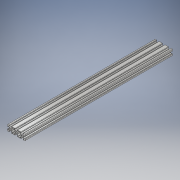
# Autodesk Inventor part: Aluminium Profile 2060 500mm
Saved by Autodesk Inventor 2019 (Build 230136000, 136)
## iProperties
Created: 2020-11-22
Part Number: Aluminium Profile 2060 500mm
Material: Aluminum 6061
Document SubType Name: Modeling
Designer: asus
Density: 2.7 g/cm^3
Appearance: Aluminum - Polished
Author: asus
Autodesk Inventor part; units mm, degrees
ref_plane "YZ Plane" through (0, 0, 0) normal (1, 0, 0) x (0, 1, 0)
ref_plane "XZ Plane" through (0, 0, 0) normal (0, 1, 0) x (-1, 0, 0)
ref_plane "XY Plane" through (0, 0, 0) normal (0, 0, 1) x (1, 0, 0)
sketch "Sketch1" plane through (0, 0, 0) normal (0, 0, 1) x (1, 0, 0)
  line L0 (-33.69, 10) -> (-33.9, 10.21)
  line L1 (-33.9, 10.21) -> (-33.9, 12.8393)
  line L2 (-33.9, 12.8393) -> (-36.5607, 15.5)
  line L3 (-36.5607, 15.5) -> (-38.2, 15.5)
  line L4 (-38.2, 15.5) -> (-38.2, 13.395)
  line L5 (-38.2, 13.395) -> (-38.815, 13.395)
  line L6 (-38.815, 13.395) -> (-40, 14.58)
  line L7 (-40, 14.58) -> (-40, 18.5)
  arc A0 (-38.5, 20) -> (-40, 18.5) centre (-38.5, 18.5) ccw
  line L8 (-38.5, 20) -> (-34.58, 20)
  line L9 (-34.58, 20) -> (-33.395, 18.815)
  line L10 (-33.395, 18.815) -> (-33.395, 18.2)
  line L11 (-33.395, 18.2) -> (-35.5, 18.2)
  line L12 (-35.5, 18.2) -> (-35.5, 16.5607)
  line L13 (-35.5, 16.5607) -> (-32.8393, 13.9)
  line L14 (-32.8393, 13.9) -> (-30.21, 13.9)
  line L15 (-30.21, 13.9) -> (-30, 13.69)
  line L16 (-30, 13.69) -> (-29.79, 13.9)
  line L17 (-29.79, 13.9) -> (-27.1607, 13.9)
  line L18 (-27.1607, 13.9) -> (-24.5, 16.5607)
  line L19 (-24.5, 16.5607) -> (-24.5, 18.2)
  line L20 (-24.5, 18.2) -> (-26.605, 18.2)
  line L21 (-26.605, 18.2) -> (-26.605, 18.815)
  line L22 (-26.605, 18.815) -> (-25.42, 20)
  line L23 (-25.42, 20) -> (-14.58, 20)
  line L24 (-14.58, 20) -> (-13.395, 18.815)
  line L25 (-13.395, 18.815) -> (-13.395, 18.2)
  line L26 (-13.395, 18.2) -> (-15.5, 18.2)
  line L27 (-15.5, 18.2) -> (-15.5, 16.5607)
  line L28 (-15.5, 16.5607) -> (-12.8393, 13.9)
  line L29 (-12.8393, 13.9) -> (-10.21, 13.9)
  line L30 (-10.21, 13.9) -> (-10, 13.69)
  line L31 (-17.3, 16.2393) -> (-17.3, 18.2)
  line L32 (-17.3, 18.2) -> (-22.7, 18.2)
  line L33 (-22.7, 18.2) -> (-22.7, 16.2393)
  line L34 (-22.7, 16.2393) -> (-26.1, 12.8393)
  line L35 (-26.1, 12.8393) -> (-26.1, 10)
  line L36 (-13.9, 10) -> (-13.9, 12.8393)
  line L37 (-13.9, 12.8393) -> (-17.3, 16.2393)
  circle A1 centre (-10, 10) radius 2.3
  circle A2 centre (-30, 10) radius 2.3
  line L38 (-24.5, 1.8) -> (-26.605, 1.8)
  line L39 (-24.5, 3.4393) -> (-24.5, 1.8)
  line L40 (-22.7, 3.7607) -> (-26.1, 7.1607)
  line L41 (-22.7, 1.8) -> (-22.7, 3.7607)
  line L42 (-29.79, 6.1) -> (-27.1607, 6.1)
  line L43 (-30, 6.31) -> (-29.79, 6.1)
  line L44 (-30.21, 6.1) -> (-30, 6.31)
  line L45 (-32.8393, 6.1) -> (-30.21, 6.1)
  line L46 (-33.9, 9.79) -> (-33.9, 7.1607)
  line L47 (-33.69, 10) -> (-33.9, 9.79)
  line L48 (-26.1, 7.1607) -> (-26.1, 10)
  line L49 (-27.1607, 6.1) -> (-24.5, 3.4393)
  line L50 (-13.9, 10) -> (-13.9, 7.1607)
  line L51 (-12.8393, 6.1) -> (-10.21, 6.1)
  line L52 (-10.21, 6.1) -> (-10, 6.31)
  line L53 (-33.395, 1.185) -> (-33.395, 1.8)
  line L54 (-35.5, 3.4393) -> (-32.8393, 6.1)
  line L55 (-33.395, 1.8) -> (-35.5, 1.8)
  line L56 (-35.5, 1.8) -> (-35.5, 3.4393)
  line L57 (-34.58, 0) -> (-33.395, 1.185)
  line L58 (-33.9, 7.1607) -> (-36.5607, 4.5)
  line L59 (-36.5607, 4.5) -> (-38.2, 4.5)
  line L60 (-38.2, 4.5) -> (-38.2, 6.605)
  line L61 (-38.2, 6.605) -> (-38.815, 6.605)
  line L62 (-38.815, 6.605) -> (-40, 5.42)
  line L63 (-38.5, 0) -> (-34.58, 0)
  arc A3 (-40, 1.5) -> (-38.5, 0) centre (-38.5, 1.5) ccw
  line L64 (-40, 5.42) -> (-40, 1.5)
  line L65 (-26.605, 1.8) -> (-26.605, 1.185)
  line L66 (-13.9, 7.1607) -> (-17.3, 3.7607)
  line L67 (-13.395, 1.8) -> (-15.5, 1.8)
  line L68 (-17.3, 3.7607) -> (-17.3, 1.8)
  line L69 (-15.5, 1.8) -> (-15.5, 3.4393)
  line L70 (-13.395, 1.185) -> (-13.395, 1.8)
  line L71 (-14.58, 0) -> (-13.395, 1.185)
  line L72 (-17.3, 1.8) -> (-22.7, 1.8)
  line L73 (-25.42, 0) -> (-14.58, 0)
  line L74 (-26.605, 1.185) -> (-25.42, 0)
  line L75 (-15.5, 3.4393) -> (-12.8393, 6.1)
  line L76 (4.5, 18.2) -> (6.605, 18.2)
  line L77 (4.5, 16.5607) -> (4.5, 18.2)
  line L78 (2.7, 16.2393) -> (6.1, 12.8393)
  line L79 (2.7, 18.2) -> (2.7, 16.2393)
  line L80 (9.79, 13.9) -> (7.1607, 13.9)
  line L81 (10, 13.69) -> (9.79, 13.9)
  line L82 (10.21, 13.9) -> (10, 13.69)
  line L83 (12.8393, 13.9) -> (10.21, 13.9)
  line L84 (13.9, 10.21) -> (13.9, 12.8393)
  line L85 (13.69, 10) -> (13.9, 10.21)
  line L86 (6.1, 12.8393) -> (6.1, 10)
  circle A4 centre (10, 10) radius 2.3
  line L87 (7.1607, 13.9) -> (4.5, 16.5607)
  line L88 (-6.1, 10) -> (-6.1, 12.8393)
  line L89 (-7.1607, 13.9) -> (-9.79, 13.9)
  line L90 (-9.79, 13.9) -> (-10, 13.69)
  line L91 (13.395, 18.815) -> (13.395, 18.2)
  line L92 (15.5, 16.5607) -> (12.8393, 13.9)
  line L93 (13.395, 18.2) -> (15.5, 18.2)
  line L94 (15.5, 18.2) -> (15.5, 16.5607)
  line L95 (14.58, 20) -> (13.395, 18.815)
  line L96 (13.9, 12.8393) -> (16.5607, 15.5)
  line L97 (16.5607, 15.5) -> (18.2, 15.5)
  line L98 (18.2, 15.5) -> (18.2, 13.395)
  line L99 (18.2, 13.395) -> (18.815, 13.395)
  line L100 (18.815, 13.395) -> (20, 14.58)
  line L101 (18.5, 20) -> (14.58, 20)
  arc A5 (20, 18.5) -> (18.5, 20) centre (18.5, 18.5) ccw
  line L102 (20, 14.58) -> (20, 18.5)
  line L103 (6.605, 18.2) -> (6.605, 18.815)
  line L104 (-6.1, 12.8393) -> (-2.7, 16.2393)
  line L105 (-6.605, 18.2) -> (-4.5, 18.2)
  line L106 (-2.7, 16.2393) -> (-2.7, 18.2)
  line L107 (-4.5, 18.2) -> (-4.5, 16.5607)
  line L108 (-6.605, 18.815) -> (-6.605, 18.2)
  line L109 (-5.42, 20) -> (-6.605, 18.815)
  line L110 (-2.7, 18.2) -> (2.7, 18.2)
  line L111 (5.42, 20) -> (-5.42, 20)
  line L112 (6.605, 18.815) -> (5.42, 20)
  line L113 (-4.5, 16.5607) -> (-7.1607, 13.9)
  line L114 (4.5, 1.8) -> (6.605, 1.8)
  line L115 (4.5, 3.4393) -> (4.5, 1.8)
  line L116 (2.7, 3.7607) -> (6.1, 7.1607)
  line L117 (2.7, 1.8) -> (2.7, 3.7607)
  line L118 (-6.605, 1.185) -> (-6.605, 1.8)
  line L119 (-6.1, 10) -> (-6.1, 7.1607)
  line L120 (-5.42, 0) -> (-6.605, 1.185)
  line L121 (-4.5, 3.4393) -> (-7.1607, 6.1)
  line L122 (-6.605, 1.8) -> (-4.5, 1.8)
  line L123 (-4.5, 1.8) -> (-4.5, 3.4393)
  line L124 (-6.1, 7.1607) -> (-2.7, 3.7607)
  line L125 (-2.7, 1.8) -> (2.7, 1.8)
  line L126 (5.42, 0) -> (-5.42, 0)
  line L127 (-2.7, 3.7607) -> (-2.7, 1.8)
  line L128 (6.1, 7.1607) -> (6.1, 10)
  line L129 (9.79, 6.1) -> (7.1607, 6.1)
  line L130 (10, 6.31) -> (9.79, 6.1)
  line L131 (10.21, 6.1) -> (10, 6.31)
  line L132 (7.1607, 6.1) -> (4.5, 3.4393)
  line L133 (-7.1607, 6.1) -> (-9.79, 6.1)
  line L134 (-9.79, 6.1) -> (-10, 6.31)
  line L135 (13.395, 1.185) -> (13.395, 1.8)
  line L136 (12.8393, 6.1) -> (10.21, 6.1)
  line L137 (13.9, 9.79) -> (13.9, 7.1607)
  line L138 (13.69, 10) -> (13.9, 9.79)
  line L139 (15.5, 3.4393) -> (12.8393, 6.1)
  line L140 (13.395, 1.8) -> (15.5, 1.8)
  line L141 (15.5, 1.8) -> (15.5, 3.4393)
  line L142 (14.58, 0) -> (13.395, 1.185)
  line L143 (6.605, 1.8) -> (6.605, 1.185)
  line L144 (13.9, 7.1607) -> (16.5607, 4.5)
  line L145 (16.5607, 4.5) -> (18.2, 4.5)
  line L146 (18.2, 4.5) -> (18.2, 6.605)
  line L147 (18.2, 6.605) -> (18.815, 6.605)
  line L148 (18.5, 0) -> (14.58, 0)
  line L149 (18.815, 6.605) -> (20, 5.42)
  line L150 (20, 5.42) -> (20, 1.5)
  arc A6 (18.5, 0) -> (20, 1.5) centre (18.5, 1.5) ccw
  line L151 (6.605, 1.185) -> (5.42, 0)
  constraints: 304 end point, 8 point on circle, 7 centre point
extrude "Extrusion4" add sketch "Sketch1" along normal blind 500
body "Solid4"
